Autodesk Inventor part; units mm, degrees
(part 2 of 2)
sketch "スケッチ11" plane through (0, 26.2, 0) normal (0, 1, 0) x (1, 0, 0)
  arc A0 (-7.9995, 0.0868) -> (-7.9995, -0.0868) centre (0, 0) ccw
  arc A1 (-7.8748, 0.05) -> (-7.8748, -0.05) centre (0, 0) ccw
  line L0 (-7.8748, -0.05) -> (-7.9995, -0.0868)
  arc A2 (-7.9995, 0.0868) -> (-7.9995, -0.0868) centre (0, 0) ccw
  line L1 (-7.8748, 0.05) -> (-7.9995, 0.0868)
  line L2 (-7.901, 0) -> (0, 0)
  line L3 (-7.8522, -0.5992) -> (-7.974, -0.6446)
  arc A3 (-7.9861, -0.4714) -> (-7.974, -0.6446) centre (0, 0) ccw
  line L4 (-7.8591, -0.4994) -> (-7.9861, -0.4714)
  arc A4 (-7.8591, -0.4994) -> (-7.8522, -0.5992) centre (0, 0) ccw
  line L5 (-7.7912, -1.1455) -> (-7.9096, -1.1993)
  arc A5 (-7.9338, -1.0274) -> (-7.9096, -1.1993) centre (0, 0) ccw
  line L6 (-7.8052, -1.0465) -> (-7.9338, -1.0274)
  arc A6 (-7.8052, -1.0465) -> (-7.7912, -1.1455) centre (0, 0) ccw
  line L7 (-7.6924, -1.6862) -> (-7.8067, -1.7481)
  arc A7 (-7.8428, -1.5783) -> (-7.8067, -1.7481) centre (0, 0) ccw
  line L8 (-7.7132, -1.5884) -> (-7.8428, -1.5783)
  arc A8 (-7.7132, -1.5884) -> (-7.6924, -1.6862) centre (0, 0) ccw
  line L9 (-7.556, -2.2187) -> (-7.6657, -2.2884)
  arc A9 (-7.7136, -2.1215) -> (-7.6657, -2.2884) centre (0, 0) ccw
  line L10 (-7.5836, -2.1225) -> (-7.7136, -2.1215)
  arc A10 (-7.5836, -2.1225) -> (-7.556, -2.2187) centre (0, 0) ccw
  line L11 (-7.3828, -2.7403) -> (-7.4874, -2.8175)
  arc A11 (-7.5468, -2.6545) -> (-7.4874, -2.8175) centre (0, 0) ccw
  line L12 (-7.417, -2.6464) -> (-7.5468, -2.6545)
  arc A12 (-7.417, -2.6464) -> (-7.3828, -2.7403) centre (0, 0) ccw
  line L13 (-7.1737, -3.2487) -> (-7.2726, -3.333)
  arc A13 (-7.3432, -3.1744) -> (-7.2726, -3.333) centre (0, 0) ccw
  line L14 (-7.2144, -3.1573) -> (-7.3432, -3.1744)
  arc A14 (-7.2144, -3.1573) -> (-7.1737, -3.2487) centre (0, 0) ccw
  line L15 (-6.9296, -3.7412) -> (-7.0224, -3.8322)
  arc A15 (-7.1039, -3.6789) -> (-7.0224, -3.8322) centre (0, 0) ccw
  line L16 (-6.9765, -3.6529) -> (-7.1039, -3.6789)
  arc A16 (-6.9765, -3.6529) -> (-6.9296, -3.7412) centre (0, 0) ccw
  line L17 (-6.6517, -4.2154) -> (-6.738, -4.3127)
  arc A17 (-6.83, -4.1655) -> (-6.738, -4.3127) centre (0, 0) ccw
  line L18 (-6.7047, -4.1306) -> (-6.83, -4.1655)
  arc A18 (-6.7047, -4.1306) -> (-6.6517, -4.2154) centre (0, 0) ccw
  line L19 (-6.3415, -4.6692) -> (-6.4207, -4.7722)
  arc A19 (-6.5228, -4.6318) -> (-6.4207, -4.7722) centre (0, 0) ccw
  line L20 (-6.4003, -4.5883) -> (-6.5228, -4.6318)
  arc A20 (-6.4003, -4.5883) -> (-6.3415, -4.6692) centre (0, 0) ccw
  line L21 (-6.0003, -5.1002) -> (-6.0722, -5.2085)
  arc A21 (-6.1838, -5.0755) -> (-6.0722, -5.2085) centre (0, 0) ccw
  line L22 (-6.0646, -5.0235) -> (-6.1838, -5.0755)
  arc A22 (-6.0646, -5.0235) -> (-6.0003, -5.1002) centre (0, 0) ccw
  line L23 (-5.63, -5.5063) -> (-5.6941, -5.6194)
  arc A23 (-5.8147, -5.4945) -> (-5.6941, -5.6194) centre (0, 0) ccw
  line L24 (-5.6994, -5.4344) -> (-5.8147, -5.4945)
  arc A24 (-5.6994, -5.4344) -> (-5.63, -5.5063) centre (0, 0) ccw
  line L25 (-5.2321, -5.8856) -> (-5.2882, -6.0029)
  arc A25 (-5.4172, -5.8867) -> (-5.2882, -6.0029) centre (0, 0) ccw
  line L26 (-5.3065, -5.8187) -> (-5.4172, -5.8867)
  arc A26 (-5.3065, -5.8187) -> (-5.2321, -5.8856) centre (0, 0) ccw
  line L27 (-4.8088, -6.2362) -> (-4.8566, -6.3571)
  arc A27 (-4.9934, -6.2503) -> (-4.8566, -6.3571) centre (0, 0) ccw
  line L28 (-4.8876, -6.1747) -> (-4.9934, -6.2503)
  arc A28 (-4.8876, -6.1747) -> (-4.8088, -6.2362) centre (0, 0) ccw
  line L29 (-4.3621, -6.5565) -> (-4.4013, -6.6804)
  arc A29 (-4.5452, -6.5834) -> (-4.4013, -6.6804) centre (0, 0) ccw
  line L30 (-4.445, -6.5006) -> (-4.5452, -6.5834)
  arc A30 (-4.445, -6.5006) -> (-4.3621, -6.5565) centre (0, 0) ccw
  line L31 (-3.8941, -6.8448) -> (-3.9246, -6.9712)
  arc A31 (-4.0749, -6.8844) -> (-3.9246, -6.9712) centre (0, 0) ccw
  line L32 (-3.9807, -6.7948) -> (-4.0749, -6.8844)
  arc A32 (-3.9807, -6.7948) -> (-3.8941, -6.8448) centre (0, 0) ccw
  line L33 (-3.4072, -7.0998) -> (-3.4288, -7.228)
  arc A33 (-3.5848, -7.1519) -> (-3.4288, -7.228) centre (0, 0) ccw
  line L34 (-3.497, -7.0559) -> (-3.5848, -7.1519)
  arc A34 (-3.497, -7.0559) -> (-3.4072, -7.0998) centre (0, 0) ccw
  line L35 (-2.9036, -7.3202) -> (-2.9162, -7.4495)
  arc A35 (-3.0771, -7.3845) -> (-2.9162, -7.4495) centre (0, 0) ccw
  line L36 (-2.9963, -7.2827) -> (-3.0771, -7.3845)
  arc A36 (-2.9963, -7.2827) -> (-2.9036, -7.3202) centre (0, 0) ccw
  line L37 (-2.3859, -7.5049) -> (-2.3895, -7.6348)
  arc A37 (-2.5545, -7.5812) -> (-2.3895, -7.6348) centre (0, 0) ccw
  line L38 (-2.481, -7.474) -> (-2.5545, -7.5812)
  arc A38 (-2.481, -7.474) -> (-2.3859, -7.5049) centre (0, 0) ccw
  line L39 (-1.8566, -7.653) -> (-1.8511, -7.7829)
  arc A39 (-2.0195, -7.7409) -> (-1.8511, -7.7829) centre (0, 0) ccw
  line L40 (-1.9536, -7.6288) -> (-2.0195, -7.7409)
  arc A40 (-1.9536, -7.6288) -> (-1.8566, -7.653) centre (0, 0) ccw
  line L41 (-1.3182, -7.7639) -> (-1.3036, -7.8931)
  arc A41 (-1.4746, -7.8629) -> (-1.3036, -7.8931) centre (0, 0) ccw
  line L42 (-1.4167, -7.7465) -> (-1.4746, -7.8629)
  arc A42 (-1.4167, -7.7465) -> (-1.3182, -7.7639) centre (0, 0) ccw
  line L43 (-0.7734, -7.8369) -> (-0.7499, -7.9648)
  arc A43 (-0.9225, -7.9466) -> (-0.7499, -7.9648) centre (0, 0) ccw
  line L44 (-0.8729, -7.8265) -> (-0.9225, -7.9466)
  arc A44 (-0.8729, -7.8265) -> (-0.7734, -7.8369) centre (0, 0) ccw
  line L45 (-0.2249, -7.8718) -> (-0.1925, -7.9977)
  arc A45 (-0.3659, -7.9916) -> (-0.1925, -7.9977) centre (0, 0) ccw
  line L46 (-0.3248, -7.8683) -> (-0.3659, -7.9916)
  arc A46 (-0.3248, -7.8683) -> (-0.2249, -7.8718) centre (0, 0) ccw
  line L47 (0.3248, -7.8683) -> (0.3659, -7.9916)
  arc A47 (0.1925, -7.9977) -> (0.3659, -7.9916) centre (0, 0) ccw
  line L48 (0.2249, -7.8718) -> (0.1925, -7.9977)
  arc A48 (0.2249, -7.8718) -> (0.3248, -7.8683) centre (0, 0) ccw
  line L49 (0.8729, -7.8265) -> (0.9225, -7.9466)
  arc A49 (0.7499, -7.9648) -> (0.9225, -7.9466) centre (0, 0) ccw
  line L50 (0.7734, -7.8369) -> (0.7499, -7.9648)
  arc A50 (0.7734, -7.8369) -> (0.8729, -7.8265) centre (0, 0) ccw
  line L51 (1.4167, -7.7465) -> (1.4746, -7.8629)
  arc A51 (1.3036, -7.8931) -> (1.4746, -7.8629) centre (0, 0) ccw
  line L52 (1.3182, -7.7639) -> (1.3036, -7.8931)
  arc A52 (1.3182, -7.7639) -> (1.4167, -7.7465) centre (0, 0) ccw
  line L53 (1.9536, -7.6288) -> (2.0195, -7.7409)
  arc A53 (1.8511, -7.7829) -> (2.0195, -7.7409) centre (0, 0) ccw
  line L54 (1.8566, -7.653) -> (1.8511, -7.7829)
  arc A54 (1.8566, -7.653) -> (1.9536, -7.6288) centre (0, 0) ccw
  line L55 (2.481, -7.474) -> (2.5545, -7.5812)
  arc A55 (2.3895, -7.6348) -> (2.5545, -7.5812) centre (0, 0) ccw
  line L56 (2.3859, -7.5049) -> (2.3895, -7.6348)
  arc A56 (2.3859, -7.5049) -> (2.481, -7.474) centre (0, 0) ccw
  line L57 (2.9963, -7.2827) -> (3.0771, -7.3845)
  arc A57 (2.9162, -7.4495) -> (3.0771, -7.3845) centre (0, 0) ccw
  line L58 (2.9036, -7.3202) -> (2.9162, -7.4495)
  arc A58 (2.9036, -7.3202) -> (2.9963, -7.2827) centre (0, 0) ccw
  line L59 (3.497, -7.0559) -> (3.5848, -7.1519)
  arc A59 (3.4288, -7.228) -> (3.5848, -7.1519) centre (0, 0) ccw
  line L60 (3.4072, -7.0998) -> (3.4288, -7.228)
  arc A60 (3.4072, -7.0998) -> (3.497, -7.0559) centre (0, 0) ccw
  line L61 (3.9807, -6.7948) -> (4.0749, -6.8844)
  arc A61 (3.9246, -6.9712) -> (4.0749, -6.8844) centre (0, 0) ccw
  line L62 (3.8941, -6.8448) -> (3.9246, -6.9712)
  arc A62 (3.8941, -6.8448) -> (3.9807, -6.7948) centre (0, 0) ccw
  line L63 (4.445, -6.5006) -> (4.5452, -6.5834)
  arc A63 (4.4013, -6.6804) -> (4.5452, -6.5834) centre (0, 0) ccw
  line L64 (4.3621, -6.5565) -> (4.4013, -6.6804)
  arc A64 (4.3621, -6.5565) -> (4.445, -6.5006) centre (0, 0) ccw
  line L65 (4.8876, -6.1747) -> (4.9934, -6.2503)
  arc A65 (4.8566, -6.3571) -> (4.9934, -6.2503) centre (0, 0) ccw
  line L66 (4.8088, -6.2362) -> (4.8566, -6.3571)
  arc A66 (4.8088, -6.2362) -> (4.8876, -6.1747) centre (0, 0) ccw
  line L67 (5.3065, -5.8187) -> (5.4172, -5.8867)
  arc A67 (5.2882, -6.0029) -> (5.4172, -5.8867) centre (0, 0) ccw
  line L68 (5.2321, -5.8856) -> (5.2882, -6.0029)
  arc A68 (5.2321, -5.8856) -> (5.3065, -5.8187) centre (0, 0) ccw
  line L69 (5.6994, -5.4344) -> (5.8147, -5.4945)
  arc A69 (5.6941, -5.6194) -> (5.8147, -5.4945) centre (0, 0) ccw
  line L70 (5.63, -5.5063) -> (5.6941, -5.6194)
  arc A70 (5.63, -5.5063) -> (5.6994, -5.4344) centre (0, 0) ccw
  line L71 (6.0646, -5.0235) -> (6.1838, -5.0755)
  arc A71 (6.0722, -5.2085) -> (6.1838, -5.0755) centre (0, 0) ccw
  line L72 (6.0003, -5.1002) -> (6.0722, -5.2085)
  arc A72 (6.0003, -5.1002) -> (6.0646, -5.0235) centre (0, 0) ccw
  line L73 (6.4003, -4.5883) -> (6.5228, -4.6318)
  arc A73 (6.4207, -4.7722) -> (6.5228, -4.6318) centre (0, 0) ccw
  line L74 (6.3415, -4.6692) -> (6.4207, -4.7722)
  arc A74 (6.3415, -4.6692) -> (6.4003, -4.5883) centre (0, 0) ccw
  line L75 (6.7047, -4.1306) -> (6.83, -4.1655)
  arc A75 (6.738, -4.3127) -> (6.83, -4.1655) centre (0, 0) ccw
  line L76 (6.6517, -4.2154) -> (6.738, -4.3127)
  arc A76 (6.6517, -4.2154) -> (6.7047, -4.1306) centre (0, 0) ccw
  line L77 (6.9765, -3.6529) -> (7.1039, -3.6789)
  arc A77 (7.0224, -3.8322) -> (7.1039, -3.6789) centre (0, 0) ccw
  line L78 (6.9296, -3.7412) -> (7.0224, -3.8322)
  arc A78 (6.9296, -3.7412) -> (6.9765, -3.6529) centre (0, 0) ccw
  line L79 (7.2144, -3.1573) -> (7.3432, -3.1744)
  arc A79 (7.2726, -3.333) -> (7.3432, -3.1744) centre (0, 0) ccw
  line L80 (7.1737, -3.2487) -> (7.2726, -3.333)
  arc A80 (7.1737, -3.2487) -> (7.2144, -3.1573) centre (0, 0) ccw
  line L81 (7.417, -2.6464) -> (7.5468, -2.6545)
  arc A81 (7.4874, -2.8175) -> (7.5468, -2.6545) centre (0, 0) ccw
  line L82 (7.3828, -2.7403) -> (7.4874, -2.8175)
  arc A82 (7.3828, -2.7403) -> (7.417, -2.6464) centre (0, 0) ccw
  line L83 (7.5836, -2.1225) -> (7.7136, -2.1215)
  arc A83 (7.6657, -2.2884) -> (7.7136, -2.1215) centre (0, 0) ccw
  line L84 (7.556, -2.2187) -> (7.6657, -2.2884)
  arc A84 (7.556, -2.2187) -> (7.5836, -2.1225) centre (0, 0) ccw
  line L85 (7.7132, -1.5884) -> (7.8428, -1.5783)
  arc A85 (7.8067, -1.7481) -> (7.8428, -1.5783) centre (0, 0) ccw
  line L86 (7.6924, -1.6862) -> (7.8067, -1.7481)
  arc A86 (7.6924, -1.6862) -> (7.7132, -1.5884) centre (0, 0) ccw
  line L87 (7.8052, -1.0465) -> (7.9338, -1.0274)
  arc A87 (7.9096, -1.1993) -> (7.9338, -1.0274) centre (0, 0) ccw
  line L88 (7.7912, -1.1455) -> (7.9096, -1.1993)
  arc A88 (7.7912, -1.1455) -> (7.8052, -1.0465) centre (0, 0) ccw
  line L89 (7.8591, -0.4994) -> (7.9861, -0.4714)
  arc A89 (7.974, -0.6446) -> (7.9861, -0.4714) centre (0, 0) ccw
  line L90 (7.8522, -0.5992) -> (7.974, -0.6446)
  arc A90 (7.8522, -0.5992) -> (7.8591, -0.4994) centre (0, 0) ccw
  line L91 (7.8748, 0.05) -> (7.9995, 0.0868)
  arc A91 (7.9995, -0.0868) -> (7.9995, 0.0868) centre (0, 0) ccw
  line L92 (7.8748, -0.05) -> (7.9995, -0.0868)
  arc A92 (7.8748, -0.05) -> (7.8748, 0.05) centre (0, 0) ccw
  line L93 (7.8522, 0.5992) -> (7.974, 0.6446)
  arc A93 (7.9861, 0.4714) -> (7.974, 0.6446) centre (0, 0) ccw
  line L94 (7.8591, 0.4994) -> (7.9861, 0.4714)
  arc A94 (7.8591, 0.4994) -> (7.8522, 0.5992) centre (0, 0) ccw
  line L95 (7.7912, 1.1455) -> (7.9096, 1.1993)
  arc A95 (7.9338, 1.0274) -> (7.9096, 1.1993) centre (0, 0) ccw
  line L96 (7.8052, 1.0465) -> (7.9338, 1.0274)
  arc A96 (7.8052, 1.0465) -> (7.7912, 1.1455) centre (0, 0) ccw
  line L97 (7.6924, 1.6862) -> (7.8067, 1.7481)
  arc A97 (7.8428, 1.5783) -> (7.8067, 1.7481) centre (0, 0) ccw
  line L98 (7.7132, 1.5884) -> (7.8428, 1.5783)
  arc A98 (7.7132, 1.5884) -> (7.6924, 1.6862) centre (0, 0) ccw
  line L99 (7.556, 2.2187) -> (7.6657, 2.2884)
  arc A99 (7.7136, 2.1215) -> (7.6657, 2.2884) centre (0, 0) ccw
  line L100 (7.5836, 2.1225) -> (7.7136, 2.1215)
  arc A100 (7.5836, 2.1225) -> (7.556, 2.2187) centre (0, 0) ccw
  line L101 (7.3828, 2.7403) -> (7.4874, 2.8175)
  arc A101 (7.5468, 2.6545) -> (7.4874, 2.8175) centre (0, 0) ccw
  line L102 (7.417, 2.6464) -> (7.5468, 2.6545)
  arc A102 (7.417, 2.6464) -> (7.3828, 2.7403) centre (0, 0) ccw
  line L103 (7.1737, 3.2487) -> (7.2726, 3.333)
  arc A103 (7.3432, 3.1744) -> (7.2726, 3.333) centre (0, 0) ccw
  line L104 (7.2144, 3.1573) -> (7.3432, 3.1744)
  arc A104 (7.2144, 3.1573) -> (7.1737, 3.2487) centre (0, 0) ccw
  line L105 (6.9296, 3.7412) -> (7.0224, 3.8322)
  arc A105 (7.1039, 3.6789) -> (7.0224, 3.8322) centre (0, 0) ccw
  line L106 (6.9765, 3.6529) -> (7.1039, 3.6789)
  arc A106 (6.9765, 3.6529) -> (6.9296, 3.7412) centre (0, 0) ccw
  line L107 (6.6517, 4.2154) -> (6.738, 4.3127)
  arc A107 (6.83, 4.1655) -> (6.738, 4.3127) centre (0, 0) ccw
  line L108 (6.7047, 4.1306) -> (6.83, 4.1655)
  arc A108 (6.7047, 4.1306) -> (6.6517, 4.2154) centre (0, 0) ccw
  line L109 (6.3415, 4.6692) -> (6.4207, 4.7722)
  arc A109 (6.5228, 4.6318) -> (6.4207, 4.7722) centre (0, 0) ccw
  line L110 (6.4003, 4.5883) -> (6.5228, 4.6318)
  arc A110 (6.4003, 4.5883) -> (6.3415, 4.6692) centre (0, 0) ccw
  line L111 (6.0003, 5.1002) -> (6.0722, 5.2085)
  arc A111 (6.1838, 5.0755) -> (6.0722, 5.2085) centre (0, 0) ccw
  line L112 (6.0646, 5.0235) -> (6.1838, 5.0755)
  arc A112 (6.0646, 5.0235) -> (6.0003, 5.1002) centre (0, 0) ccw
  line L113 (5.63, 5.5063) -> (5.6941, 5.6194)
  arc A113 (5.8147, 5.4945) -> (5.6941, 5.6194) centre (0, 0) ccw
  line L114 (5.6994, 5.4344) -> (5.8147, 5.4945)
  arc A114 (5.6994, 5.4344) -> (5.63, 5.5063) centre (0, 0) ccw
  line L115 (5.2321, 5.8856) -> (5.2882, 6.0029)
  arc A115 (5.4172, 5.8867) -> (5.2882, 6.0029) centre (0, 0) ccw
  line L116 (5.3065, 5.8187) -> (5.4172, 5.8867)
  arc A116 (5.3065, 5.8187) -> (5.2321, 5.8856) centre (0, 0) ccw
  line L117 (4.8088, 6.2362) -> (4.8566, 6.3571)
  arc A117 (4.9934, 6.2503) -> (4.8566, 6.3571) centre (0, 0) ccw
  line L118 (4.8876, 6.1747) -> (4.9934, 6.2503)
  arc A118 (4.8876, 6.1747) -> (4.8088, 6.2362) centre (0, 0) ccw
  line L119 (4.3621, 6.5565) -> (4.4013, 6.6804)
  arc A119 (4.5452, 6.5834) -> (4.4013, 6.6804) centre (0, 0) ccw
  line L120 (4.445, 6.5006) -> (4.5452, 6.5834)
  arc A120 (4.445, 6.5006) -> (4.3621, 6.5565) centre (0, 0) ccw
  line L121 (3.8941, 6.8448) -> (3.9246, 6.9712)
  arc A121 (4.0749, 6.8844) -> (3.9246, 6.9712) centre (0, 0) ccw
  line L122 (3.9807, 6.7948) -> (4.0749, 6.8844)
  arc A122 (3.9807, 6.7948) -> (3.8941, 6.8448) centre (0, 0) ccw
  line L123 (3.4072, 7.0998) -> (3.4288, 7.228)
  arc A123 (3.5848, 7.1519) -> (3.4288, 7.228) centre (0, 0) ccw
  line L124 (3.497, 7.0559) -> (3.5848, 7.1519)
  arc A124 (3.497, 7.0559) -> (3.4072, 7.0998) centre (0, 0) ccw
  line L125 (2.9036, 7.3202) -> (2.9162, 7.4495)
  arc A125 (3.0771, 7.3845) -> (2.9162, 7.4495) centre (0, 0) ccw
  line L126 (2.9963, 7.2827) -> (3.0771, 7.3845)
  arc A126 (2.9963, 7.2827) -> (2.9036, 7.3202) centre (0, 0) ccw
  line L127 (2.3859, 7.5049) -> (2.3895, 7.6348)
  arc A127 (2.5545, 7.5812) -> (2.3895, 7.6348) centre (0, 0) ccw
  line L128 (2.481, 7.474) -> (2.5545, 7.5812)
  arc A128 (2.481, 7.474) -> (2.3859, 7.5049) centre (0, 0) ccw
  line L129 (1.8566, 7.653) -> (1.8511, 7.7829)
  arc A129 (2.0195, 7.7409) -> (1.8511, 7.7829) centre (0, 0) ccw
  line L130 (1.9536, 7.6288) -> (2.0195, 7.7409)
  arc A130 (1.9536, 7.6288) -> (1.8566, 7.653) centre (0, 0) ccw
  line L131 (1.3182, 7.7639) -> (1.3036, 7.8931)
  arc A131 (1.4746, 7.8629) -> (1.3036, 7.8931) centre (0, 0) ccw
  line L132 (1.4167, 7.7465) -> (1.4746, 7.8629)
  arc A132 (1.4167, 7.7465) -> (1.3182, 7.7639) centre (0, 0) ccw
  line L133 (0.7734, 7.8369) -> (0.7499, 7.9648)
  arc A133 (0.9225, 7.9466) -> (0.7499, 7.9648) centre (0, 0) ccw
  line L134 (0.8729, 7.8265) -> (0.9225, 7.9466)
  arc A134 (0.8729, 7.8265) -> (0.7734, 7.8369) centre (0, 0) ccw
  line L135 (0.2249, 7.8718) -> (0.1925, 7.9977)
  arc A135 (0.3659, 7.9916) -> (0.1925, 7.9977) centre (0, 0) ccw
  line L136 (0.3248, 7.8683) -> (0.3659, 7.9916)
  arc A136 (0.3248, 7.8683) -> (0.2249, 7.8718) centre (0, 0) ccw
  line L137 (-0.3248, 7.8683) -> (-0.3659, 7.9916)
  arc A137 (-0.1925, 7.9977) -> (-0.3659, 7.9916) centre (0, 0) ccw
  line L138 (-0.2249, 7.8718) -> (-0.1925, 7.9977)
  arc A138 (-0.2249, 7.8718) -> (-0.3248, 7.8683) centre (0, 0) ccw
  line L139 (-0.8729, 7.8265) -> (-0.9225, 7.9466)
  arc A139 (-0.7499, 7.9648) -> (-0.9225, 7.9466) centre (0, 0) ccw
  line L140 (-0.7734, 7.8369) -> (-0.7499, 7.9648)
  arc A140 (-0.7734, 7.8369) -> (-0.8729, 7.8265) centre (0, 0) ccw
  line L141 (-1.4167, 7.7465) -> (-1.4746, 7.8629)
  arc A141 (-1.3036, 7.8931) -> (-1.4746, 7.8629) centre (0, 0) ccw
  line L142 (-1.3182, 7.7639) -> (-1.3036, 7.8931)
  arc A142 (-1.3182, 7.7639) -> (-1.4167, 7.7465) centre (0, 0) ccw
  line L143 (-1.9536, 7.6288) -> (-2.0195, 7.7409)
  arc A143 (-1.8511, 7.7829) -> (-2.0195, 7.7409) centre (0, 0) ccw
  line L144 (-1.8566, 7.653) -> (-1.8511, 7.7829)
  arc A144 (-1.8566, 7.653) -> (-1.9536, 7.6288) centre (0, 0) ccw
  line L145 (-2.481, 7.474) -> (-2.5545, 7.5812)
  arc A145 (-2.3895, 7.6348) -> (-2.5545, 7.5812) centre (0, 0) ccw
  line L146 (-2.3859, 7.5049) -> (-2.3895, 7.6348)
  arc A146 (-2.3859, 7.5049) -> (-2.481, 7.474) centre (0, 0) ccw
  line L147 (-2.9963, 7.2827) -> (-3.0771, 7.3845)
  arc A147 (-2.9162, 7.4495) -> (-3.0771, 7.3845) centre (0, 0) ccw
  line L148 (-2.9036, 7.3202) -> (-2.9162, 7.4495)
  arc A148 (-2.9036, 7.3202) -> (-2.9963, 7.2827) centre (0, 0) ccw
  line L149 (-3.497, 7.0559) -> (-3.5848, 7.1519)
  arc A149 (-3.4288, 7.228) -> (-3.5848, 7.1519) centre (0, 0) ccw
  line L150 (-3.4072, 7.0998) -> (-3.4288, 7.228)
  arc A150 (-3.4072, 7.0998) -> (-3.497, 7.0559) centre (0, 0) ccw
  line L151 (-3.9807, 6.7948) -> (-4.0749, 6.8844)
  arc A151 (-3.9246, 6.9712) -> (-4.0749, 6.8844) centre (0, 0) ccw
  line L152 (-3.8941, 6.8448) -> (-3.9246, 6.9712)
  arc A152 (-3.8941, 6.8448) -> (-3.9807, 6.7948) centre (0, 0) ccw
  line L153 (-4.445, 6.5006) -> (-4.5452, 6.5834)
  arc A153 (-4.4013, 6.6804) -> (-4.5452, 6.5834) centre (0, 0) ccw
  line L154 (-4.3621, 6.5565) -> (-4.4013, 6.6804)
  arc A154 (-4.3621, 6.5565) -> (-4.445, 6.5006) centre (0, 0) ccw
  line L155 (-4.8876, 6.1747) -> (-4.9934, 6.2503)
  arc A155 (-4.8566, 6.3571) -> (-4.9934, 6.2503) centre (0, 0) ccw
  line L156 (-4.8088, 6.2362) -> (-4.8566, 6.3571)
  arc A156 (-4.8088, 6.2362) -> (-4.8876, 6.1747) centre (0, 0) ccw
  line L157 (-5.3065, 5.8187) -> (-5.4172, 5.8867)
  arc A157 (-5.2882, 6.0029) -> (-5.4172, 5.8867) centre (0, 0) ccw
  line L158 (-5.2321, 5.8856) -> (-5.2882, 6.0029)
  arc A158 (-5.2321, 5.8856) -> (-5.3065, 5.8187) centre (0, 0) ccw
  line L159 (-5.6994, 5.4344) -> (-5.8147, 5.4945)
  arc A159 (-5.6941, 5.6194) -> (-5.8147, 5.4945) centre (0, 0) ccw
  line L160 (-5.63, 5.5063) -> (-5.6941, 5.6194)
  arc A160 (-5.63, 5.5063) -> (-5.6994, 5.4344) centre (0, 0) ccw
  line L161 (-6.0646, 5.0235) -> (-6.1838, 5.0755)
  arc A161 (-6.0722, 5.2085) -> (-6.1838, 5.0755) centre (0, 0) ccw
  line L162 (-6.0003, 5.1002) -> (-6.0722, 5.2085)
  arc A162 (-6.0003, 5.1002) -> (-6.0646, 5.0235) centre (0, 0) ccw
  line L163 (-6.4003, 4.5883) -> (-6.5228, 4.6318)
  arc A163 (-6.4207, 4.7722) -> (-6.5228, 4.6318) centre (0, 0) ccw
  line L164 (-6.3415, 4.6692) -> (-6.4207, 4.7722)
  arc A164 (-6.3415, 4.6692) -> (-6.4003, 4.5883) centre (0, 0) ccw
  line L165 (-6.7047, 4.1306) -> (-6.83, 4.1655)
  arc A165 (-6.738, 4.3127) -> (-6.83, 4.1655) centre (0, 0) ccw
  line L166 (-6.6517, 4.2154) -> (-6.738, 4.3127)
  arc A166 (-6.6517, 4.2154) -> (-6.7047, 4.1306) centre (0, 0) ccw
  line L167 (-6.9765, 3.6529) -> (-7.1039, 3.6789)
  arc A167 (-7.0224, 3.8322) -> (-7.1039, 3.6789) centre (0, 0) ccw
  line L168 (-6.9296, 3.7412) -> (-7.0224, 3.8322)
  arc A168 (-6.9296, 3.7412) -> (-6.9765, 3.6529) centre (0, 0) ccw
  line L169 (-7.2144, 3.1573) -> (-7.3432, 3.1744)
  arc A169 (-7.2726, 3.333) -> (-7.3432, 3.1744) centre (0, 0) ccw
  line L170 (-7.1737, 3.2487) -> (-7.2726, 3.333)
  arc A170 (-7.1737, 3.2487) -> (-7.2144, 3.1573) centre (0, 0) ccw
  line L171 (-7.417, 2.6464) -> (-7.5468, 2.6545)
  arc A171 (-7.4874, 2.8175) -> (-7.5468, 2.6545) centre (0, 0) ccw
  line L172 (-7.3828, 2.7403) -> (-7.4874, 2.8175)
  arc A172 (-7.3828, 2.7403) -> (-7.417, 2.6464) centre (0, 0) ccw
  line L173 (-7.5836, 2.1225) -> (-7.7136, 2.1215)
  arc A173 (-7.6657, 2.2884) -> (-7.7136, 2.1215) centre (0, 0) ccw
  line L174 (-7.556, 2.2187) -> (-7.6657, 2.2884)
  arc A174 (-7.556, 2.2187) -> (-7.5836, 2.1225) centre (0, 0) ccw
  line L175 (-7.7132, 1.5884) -> (-7.8428, 1.5783)
  arc A175 (-7.8067, 1.7481) -> (-7.8428, 1.5783) centre (0, 0) ccw
  line L176 (-7.6924, 1.6862) -> (-7.8067, 1.7481)
  arc A176 (-7.6924, 1.6862) -> (-7.7132, 1.5884) centre (0, 0) ccw
  line L177 (-7.8052, 1.0465) -> (-7.9338, 1.0274)
  arc A177 (-7.9096, 1.1993) -> (-7.9338, 1.0274) centre (0, 0) ccw
  line L178 (-7.7912, 1.1455) -> (-7.9096, 1.1993)
  arc A178 (-7.7912, 1.1455) -> (-7.8052, 1.0465) centre (0, 0) ccw
  line L179 (-7.8591, 0.4994) -> (-7.9861, 0.4714)
  arc A179 (-7.974, 0.6446) -> (-7.9861, 0.4714) centre (0, 0) ccw
  line L180 (-7.8522, 0.5992) -> (-7.974, 0.6446)
  arc A180 (-7.8522, 0.5992) -> (-7.8591, 0.4994) centre (0, 0) ccw
  dimension "d37" = 15.75
  dimension "d38" = 0.13
  dimension "d39" = 0.13
  dimension "d40" = 0.1
  dimension "d41" = 0.05
  dimension "d42" = 360
  constraints: 362 end point, 362 point on circle, 181 centre point, 90 coincident, 1 horizontal, 902 other
  measures "d37" diameter of A1
  measures "d38" distance of L0.end L0.start
  measures "d39" distance of L1.end L1.start
  measures "d40" distance of L1.start L0.start
  measures "d41" distance from line of L2 L0.start
extrude "押し出し11" cut sketch "スケッチ11" against normal blind 1.75
fillet "フィレット1" radius 0.5 1 edges at (-6.25, 5.5, 0)
thread "ねじ2" size "M14x2" class "6g" standard "ANSI Metric M Profile" length 17 offset 0.5
